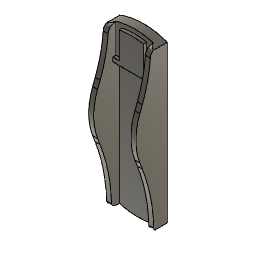
model (Autodesk Fusion 360 design; units mm, degrees)
Autodesk Fusion 360 part; units mm, degrees
sketch "sole" plane through (0, 0, 0) normal (0, 1, 0) x (1, 0, 0) in component "plane"
  line L0 (0, 0) -> (0, -147)
  line L1 (44.3, 0) -> (44.3, -147)
  arc A0 (0, -147) -> (44.3, -147) centre (22.15, -87.6722) ccw
  arc A1 (44.3, 0) -> (0, 0) centre (22.15, -59.3278) ccw
  line L2 (0, -147) -> (44.3, -147) construction
  line L3 (0, 0) -> (44.3, 0) construction
  line L4 (22.15, -147) -> (22.15, -151) construction
  line L5 (22.15, 4) -> (22.15, 0) construction
  line L6 (4.65, -148.534) -> (4.65, 1.534)
  line L7 (39.65, -148.534) -> (39.65, 1.534)
  line L8 (0, -73.5) -> (4.65, -73.5) construction
  line L9 (39.65, -73.5) -> (44.3, -73.5) construction
  line L10 (4.65, -120.9471) -> (10.65, -120.9471)
  line L11 (10.65, -120.9471) -> (10.65, -145.9471)
  arc A2 (10.65, -145.9471) -> (33.65, -145.9471) centre (22.15, -83.6722) ccw
  line L12 (33.65, -145.9471) -> (33.65, -120.9471)
  line L13 (33.65, -120.9471) -> (39.65, -120.9471)
  line L14 (4.65, -116.9471) -> (39.65, -116.9471)
  point P0 (22.15, -147)
  dimension "d17" = 4
  dimension "d18" = 44.3
  dimension "d19" = 147
  dimension "d20" = 35
  dimension "d21" = 6
  dimension "d22" = 25
  dimension "d23" = 4
  constraint coincident L0.start A1.end
  constraint vertical L0
  constraint horizontal L2
  constraint vertical L1
  constraint horizontal L3
  constraint midpoint L2 P0
  constraint midpoint A0 L4.end
  constraint midpoint A1 L5.start
  constraint midpoint L3 L5.end
  constraint equal L4 L5
  constraint coincident A0 L6.start
  constraint coincident A1 L6.end
  constraint coincident A0 L7.start
  constraint coincident A1 L7.end
  constraint vertical L6
  constraint vertical L7
  constraint midpoint L0 L8.start
  constraint midpoint L6 L8.end
  constraint midpoint L7 L9.start
  constraint midpoint L1 L9.end
  constraint equal L8 L9
  constraint coincident L6 L10.start
  constraint perpendicular L1 L10
  constraint perpendicular L10 L11
  constraint parallel L1 L12
  constraint coincident L7 L13.end
  constraint perpendicular L7 L13
  constraint equal L10 L13
  constraint equal A0 A2
  constraint midpoint A2 P0
  constraint coincident P0 L4.start
  constraint collinear L10 L13
  constraint coincident L6 L14.start
  constraint coincident L7 L14.end
  constraint perpendicular L7 L14
  measures "d17" distance of P0 L4.end
  measures "d18" distance of L0 L1
  measures "d19" distance of L0.start L0.end
  measures "d20" distance of L6 L7
  measures "d21" distance of L6 L11
  measures "d22" distance of L10.end L11.end
  measures "d23" distance of L10 L14
extrude "Extrude1" add sketch "sole" against normal blind 5 contours A1 L6 L7 L14 makes body 1 in component "plane"
extrude "Extrude2" add sketch "sole" against normal blind 8.5 separate body contours A0 L6 L7 L10 L11 A2 L12 L13 makes body 2 in component "plane"
extrude "Extrude3" add sketch "sole" against normal up to surface (11.5 mm away) contours L6 L7 L10 L11 A2 L12 L13 L14 bodies 1 2 in component "plane"
extrude "Extrude4" add sketch "sole" against normal blind 29.4 contours L0 A0 A1 L6 | L1 A0 A1 L7 bodies 1 in component "plane"
sketch "side" plane through (44.3, 0, 0) normal (1, 0, 0) x (0, 1, 0) in component "plane"
  line L0 (0, 0) -> (0, 147)
  line L1 (0, 147) -> (-29.4, 147)
  line L2 (-29.4, 147) -> (-29.4, 0)
  line L3 (-29.4, 0) -> (0, 0)
  arc A0 (-10, 148.3345) -> (-15.8788, 142.0768) centre (-9.1047, 141.6032) ccw
  arc A1 (-12.6027, 2.0001) -> (-10, -0.869) centre (-9.6045, 2.1048) ccw
  arc A2 (-12.6027, 2.0001) -> (-23.3889, 55.5396) centre (-179.8644, -3.8408) ccw
  arc A3 (-25.7327, 101.7158) -> (-25.7327, 61.7158) centre (26.97, 81.7158) ccw
  arc A4 (-23.3889, 107.8921) -> (-15.8788, 142.0768) centre (-135.5155, 150.4427) ccw
  line L4 (-25.7327, 101.7158) -> (-23.3889, 107.8921)
  line L5 (-25.7327, 61.7158) -> (-23.3889, 55.5396)
  line L6 (-10, 148.3345) -> (-10, -0.869) construction
  line L7 (-12.6027, 2.0001) -> (-15.8788, 142.0768) construction
  line L8 (-25.7327, 101.7158) -> (-25.7327, 61.7158) construction
  line L9 (-23.3889, 55.5396) -> (-23.3889, 107.8921) construction
  line L10 (-29.4, 81.7158) -> (0, 81.7158) construction
  line L11 (-10, -0.869) -> (0, -2.199)
  line L12 (-10, 148.3345) -> (0, 149.6645)
  line L13 (0, 147) -> (0, 149.6645)
  line L14 (-5, -1.534) -> (0, -2.199) construction
  line L15 (0, -2.199) -> (0, 0)
  line L16 (-15.8788, 142.0768) -> (-12.2887, 193.4184) construction
  line L17 (-12.6027, 2.0001) -> (-11.4651, -30.5765) construction
  line L18 (-8.5, 148.534) -> (-29.4, 148.534)
  line L19 (-29.4, 148.534) -> (-29.4, -1.534)
  line L20 (-29.4, -1.534) -> (-5, -1.534)
  point P0 (-8.5, 148.534)
  point P1 (-29.4, 148.534)
  point P2 (-29.4, -1.534)
  point P3 (-5, -1.534)
  dimension "d34" = 40
  dimension "d35" = 66.8182
  dimension "d36" = 10
  dimension "d38" = 1.33
  dimension "d39" = 1.33
  dimension "d40" = 3
  dimension "d42" = 35
  dimension "d43" = 4
  dimension "d45" = 2
  constraint tangent A0 A4
  constraint tangent A4 L4
  constraint tangent A3 L4
  constraint tangent A3 L5
  constraint tangent A2 L5
  constraint tangent A1 A2
  constraint vertical L8
  constraint vertical L6
  constraint vertical L9
  constraint midpoint A3 L10.start
  constraint coincident L0 L10.end
  constraint perpendicular L0 L10
  constraint coincident P3 L14.start
  constraint coincident L0.end L1.start
  constraint tangent A0 L12
  constraint tangent A1 L11
  constraint coincident L0.start L3.end
  constraint perpendicular L3 L15
  constraint coincident L11.end L14.end
  constraint coincident L2 L10.start
  constraint tangent A4 L16
  constraint tangent A1 L17
  constraint coincident P3 L11
  constraint coincident P0 L12
  constraint vertical L13
  constraint coincident P0 L18.start
  constraint coincident P1 L18.end
  constraint coincident P2 L19.end
  measures "d34" vertical distance of A3.end A3.start
  measures "d35" distance of P0 L10
  measures "d36" distance of L0 L6
  measures "d38" vertical distance of A0.start L12.end
  measures "d39" vertical distance of A1.end L11.end
  measures "d40" radius of A1
  measures "d42" distance of A0.end A4.start
  measures "d43" angle of L0 L16
  measures "d45" angle of L0 L17
extrude "Extrude5" cut sketch "side" against normal up to surface (44.3 mm away) contours L3 A1 L11 L19 L20 | L2 L3 A1 A2 A3 L5 L19 | L1 L2 A0 A3 A4 L4 L19 | L1 A0 L12 L18 L19 bodies 1 in component "plane"
component "top" placed x (1, 0, 0) y (0, 1, 0) z (0, 0, 1) at (0, 0, 0)
component "plane" placed x (1, 0, 0) y (0, 1, 0) z (0, 0, 1) at (0, 0, 0)
component "bot" placed x (1, 0, 0) y (0, 1, 0) z (0, 0, 1) at (0, 0, 0)
equation "outerWidth = 44.3 mm"
equation "innerWidth = 35 mm"
equation "frontThickness = 8.5 mm"
equation "frontHeight = 12 mm"
equation "backHeight = 13 mm"
equation "humpHeight = 29.4 mm"
equation "humpArcLength = 40 mm"
equation "frontArcLength = 35 mm"
equation "sideLength = 147 mm"
equation "soleArcProjection = 4 mm"
equation "sideAngleX = 1.33 mm"
equation "frontSlotWidth = 6 mm"
equation "backThickness = 5 mm"
equation "backMaxDepth = 7 mm"
equation "backKnobClearance = 3 mm"
equation "backKnobDiameter = 19 mm"
equation "d17 = soleArcProjection"
equation "d18 = outerWidth"
equation "d19 = sideLength"
equation "d20 = innerWidth"
equation "d21 = frontSlotWidth"
equation "d24 = -backThickness"
equation "d26 = -frontThickness"
equation "d30 = -humpHeight"
equation "d32 = sideAngleX"
equation "d34 = humpArcLength"
equation "d35 = sideLength * 5 / 11"
equation "d38 = sideAngleX"
equation "d39 = sideAngleX"
